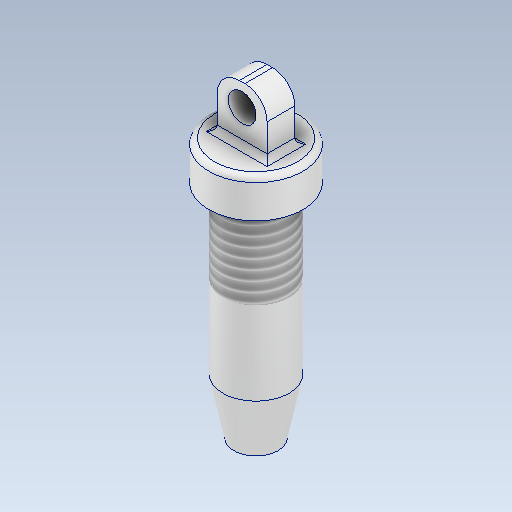
# Autodesk Inventor part: Korpus
Saved by Autodesk Inventor 2020 (Build 240168000, 168)
## iProperties
Created: 2021-03-25
Part Number: Korpus
Material: Aluminum 6061
Document SubType Name: Modeling
Designer: patry
Density: 2.7 g/cm^3
Appearance: Aluminum - Flat
Mass: 10.9517 g
Surface Area: 35.4588 cm^2
Volume: 4.05619 cm^3
Author: patry
Autodesk Inventor part; units mm, degrees
ref_plane "YZ Plane" through (0, 0, 0) normal (1, 0, 0) x (0, 1, 0)
ref_plane "XZ Plane" through (0, 0, 0) normal (0, 1, 0) x (-1, 0, 0)
ref_plane "XY Plane" through (0, 0, 0) normal (0, 0, 1) x (1, 0, 0)
sketch "Szkic1" plane through (0, 0, 0) normal (0, 1, 0) x (-1, 0, 0)
  circle A0 centre (0, 0) radius 8.5
  dimension "d0" = 17
  constraints: 1 centre point, 1 coincident
  measures "d0" diameter of A0
extrude "Wyciągnięcie proste1" add sketch "Szkic1" along normal blind 7
sketch "Szkic2" plane through (0, 7, 0) normal (0, 1, 0) x (1, 0, 0)
  line L0 (4.5, -2.5) -> (-4.5, -2.5)
  line L1 (-4.5, -2.5) -> (-4.5, 2.5)
  line L2 (-4.5, 2.5) -> (4.5, 2.5)
  line L3 (4.5, 2.5) -> (4.5, -2.5)
  line L4 (4.5, -2.5) -> (-4.5, 2.5) construction
  line L5 (-4.5, -2.5) -> (4.5, 2.5) construction
  point P0 (0, 0)
  dimension "d3" = 9
  dimension "d4" = 5
  constraints: 12 end point, 2 midpoint, 2 parallel, 1 horizontal, 1 perpendicular
  measures "d3" distance of L1.end L2.end
  measures "d4" distance of L0.end L1.end
extrude "Wyciągnięcie proste2" add sketch "Szkic2" along normal blind 10
fillet "Zaokrąglenie1" radius 4 2 edges at (4.5, 17, 0) (-4.5, 17, 0)
sketch "Szkic3" plane through (-4.5, 7, 2.5) normal (0, 0, 1) x (1, 0, 0)
  arc A0 (9, 6) -> (5, 10) centre (5, 6) ccw projected
  arc A1 (4, 10) -> (0, 6) centre (4, 6) ccw projected
  circle A2 centre (4.5, 6) radius 2.5
  point P0 (4.5, -7)
  dimension "d8" = 5
  constraints: 1 centre point, 1 coincident
  measures "d8" diameter of A2
extrude "Wyciągnięcie proste3" cut sketch "Szkic3" against normal blind 10
fillet "Zaokrąglenie2" radius 1 1 edges at (8.5, 7, 0)
fillet "Zaokrąglenie3" radius 1 4 edges at (0, 7, 2.5) (4.5, 7, 0) (0, 7, -2.5) (-4.5, 7, 0)
sketch "Szkic4" plane through (0, 0, 0) normal (0, -1, 0) x (1, 0, 0)
  circle A0 centre (0, 0) radius 6
  circle A1 centre (0, 0) radius 4.5
  dimension "d13" = 12
  dimension "d21" = 9
  constraints: 2 centre point, 2 coincident
  measures "d13" diameter of A0
  measures "d21" diameter of A1
extrude "Wyciągnięcie proste4" add sketch "Szkic4" along normal blind 30 from surface at 0
thread "Gwint1" size "M12x1.75" class "6g" standard "ANSI Metric M Profile" length 15
sketch "Szkic5" plane through (0, -30, 0) normal (0, -1, 0) x (1, 0, 0)
  circle A0 centre (0, 0) radius 2
  circle A1 centre (0, 0) radius 6
  dimension "d22" = 4
  constraints: 2 centre point, 2 coincident
  measures "d22" diameter of A0
extrude "Wyciągnięcie proste5" add sketch "Szkic5" along normal blind 10
chamfer "Faza2" distance 2 distance2 10 1 edges at (-6, -40, 0) measured on face at (4.5892, -40, -0.6382)
